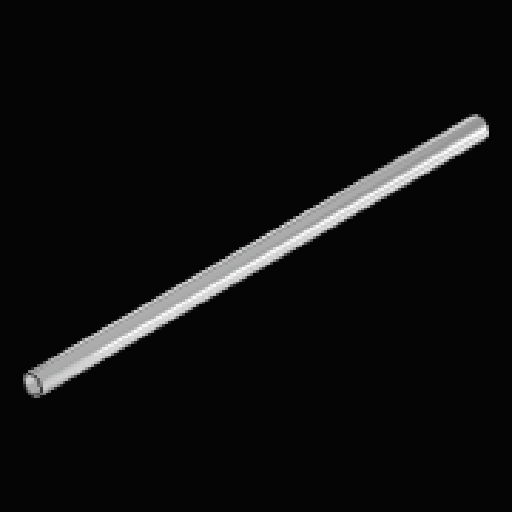
# Autodesk Inventor part: Rack Rail v3
Saved by Autodesk Inventor 2023.2 (Build 272271030, 271C)
## iProperties
Created: 2023-11-22
Part Number: Rack Rail v3
Material: Aluminum 6061
Document SubType Name: Modeling
Designer: robpl
Density: 2.7 g/cm^3
Appearance: Aluminum - Flat
Author: robpl
Autodesk Inventor part; units mm, degrees
ref_plane "YZ Plane" through (0, 0, 0) normal (1, 0, 0) x (0, 1, 0)
ref_plane "XZ Plane" through (0, 0, 0) normal (0, 1, 0) x (-1, 0, 0)
ref_plane "XY Plane" through (0, 0, 0) normal (0, 0, 1) x (1, 0, 0)
sketch "Sketch1" plane through (0, 0, 0) normal (0, 0, 1) x (1, 0, 0)
  circle A0 centre (0, 0) radius 1.9844
  circle A1 centre (0, 0) radius 1.6288
  dimension "d0" = 3.9688
  dimension "d3" = 0.3556
  constraints: 2 centre point, 1 coincident
  measures "d0" diameter of A0
  measures "d3" radial gap between concentric circles of A0 A1
extrude "Extrusion1" add sketch "Sketch1" along normal blind 90
body "Solid1"
